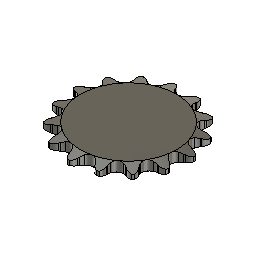
25Chain Sprocket Generator (Autodesk Fusion 360 design; units mm, degrees)
Autodesk Fusion 360 part; units mm, degrees
sketch "Teeth" plane through (0, 0, 0) normal (0, 0, 1) x (1, 0, 0)
  circle A0 centre (0, 0) radius 15.2709 construction
  line L0 (0, 15.2709) -> (-6.2112, 13.9507) construction
  arc A1 (-1.8813, 15.121) -> (-1.3133, 14.2074) centre (2.0529, 16.9333) ccw
  line L1 (-1.8813, 15.121) -> (-2.0352, 15.4552)
  arc A2 (-2.0352, 15.4552) -> (-3.2085, 16.7119) centre (-4.5218, 14.3098) ccw
  line L2 (0, 15.2709) -> (3.9262, 15.2709) construction
  line L3 (-1.8813, 15.121) -> (2.0529, 16.9333) construction
  line L4 (2.0529, 16.9333) -> (0, 15.2709) construction
  line L5 (0, 15.2709) -> (0, 0) construction
  arc A3 (-1.3133, 14.2074) -> (0, 13.581) centre (0, 15.2709) ccw
  arc A4 (3.2085, 16.7119) -> (2.0352, 15.4552) centre (4.5218, 14.3098) ccw
  line L6 (1.8813, 15.121) -> (2.0352, 15.4552)
  arc A5 (1.3133, 14.2074) -> (1.8813, 15.121) centre (-2.0529, 16.9333) ccw
  arc A6 (0, 13.581) -> (1.3133, 14.2074) centre (0, 15.2709) ccw
  arc A7 (-3.2085, 16.7119) -> (-3.5381, 16.6453) centre (0, 0) ccw
  arc A8 (3.5381, 16.6453) -> (3.2085, 16.7119) centre (0, 0) ccw
  circle A9 centre (0, 0) radius 17.0172
  dimension "d11" = 30.5418
  dimension "d12" = 6.35
  dimension "d14" = 39
  dimension "d15" = 14.267
  dimension "d16" = 2.6416
  dimension "d17" = 4.6228
  dimension "d18" = 1.6899
  dimension "d20" = 17.0172
  dimension "d50" = 34.0343
  constraint coincident A0.centre L5.end
  constraint coincident A0 L0.start
  constraint coincident A0 L0.end
  constraint vertical A0.centre L0.start
  constraint tangent A1 L1
  constraint tangent L1 A2
  constraint tangent A0 L2
  constraint horizontal L2
  constraint perpendicular L1 L3
  constraint coincident L0 A2.centre
  constraint coincident A1.centre L3.end
  constraint coincident L5 A3.end
  constraint coincident L0 L2.start
  constraint coincident L0.start L2.start
  constraint tangent A1 A3
  constraint symmetric A1.end L5 A5.start
  constraint symmetric A1.start L5 L6.start
  constraint symmetric A1 L5 A5
  constraint symmetric L1.end L5 A4.end
  constraint symmetric A2 L5 A4
  constraint symmetric L5 A3.end A6.start
  constraint symmetric L5 A3 A6
  constraint vertical A0.centre A3.end
  constraint symmetric L5 A2.end A4.start
  constraint symmetric L5 A7.end A8.start
  constraint symmetric L5 A7 A8
  constraint coincident A4.start A8.end
  measures "d11" diameter of A0
  measures "d12" distance of L0.start L0.end
  measures "d14" angle of L2 L4
  measures "d15" angle of L3 L4
  measures "d16" distance of A1.centre L0.start
  measures "d17" distance of A2.centre L0.start
  measures "d18" radius of A3
  measures "d20" radius of A7
  measures "d50" diameter of A9
extrude "Extrude1" add sketch "Teeth" along normal mid plane 2.794
extrude "Extrude3" cut sketch "Teeth" along normal through all and the other way through all contours A1 L1 A2 A3 A4 L6 A5 A6 A9
pattern_circular "C-Pattern1" count 15 over 360 about axis through (0, 0, 0) along (0, 0, 1) of "Extrude3"
sketch "Sketch4" plane through (0, 0, 0) normal (1, 0, 0) x (0, 1, 0)
  line L0 (-17.0172, 0.635) -> (-13.581, 1.397)
  line L1 (-13.581, 1.397) -> (0, 1.397)
  line L2 (-13.581, -1.397) -> (0, -1.397)
  line L3 (-17.0172, -0.635) -> (-13.581, -1.397)
  line L4 (0, 1.397) -> (0, -1.397)
  line L5 (-17.0172, 0.635) -> (-17.0172, -0.635)
  point P0 (-39.6283, 3.175)
  point P1 (-17.0172, 0)
  dimension "d54" = 2.794
  dimension "d55" = 17.0172
  dimension "d56" = 13.581
  dimension "d57" = 1.27
  constraint horizontal L1
  constraint horizontal L2
  constraint midpoint L4 origin
  constraint vertical L5
  constraint equal L1 L2
  constraint midpoint L5 P1
  constraint horizontal origin P1
  measures "d54" distance of L1.end L2.end
  measures "d55" distance of L4 L5
  measures "d56" distance of L2.end L2.start
  measures "d57" distance of L0.start L3.start
revolve "Revolve1" cut sketch "Sketch4" angle 360 about axis through (0, 0, 1.75) along (0, 0, 1) keep common part
equation "p = 0.25 in" comment "0.25 for #25, 0.375 for #35"
equation "Dr = 0.13 in" comment "0.13 for #25, 0.2 for #35"
equation "Ds = 1.0005 * Dr + 0.003 in"
equation "n = 15" comment "Number of Teeth"
equation "PD = p / sin(( 180 / n ) * 1 deg)"
equation "A_angle = 35 deg + ( 60 / n ) * 1 deg"
equation "B_angle = 18 deg - ( 56 / n ) * 1 deg"
equation "ac = 0.8 * Dr"
equation "ab = 1.4 * Dr"
equation "OD = PD + 0.55 * p"
equation "d11 = PD"
equation "d12 = p"
equation "d14 = A_angle"
equation "d15 = B_angle"
equation "d16 = ac"
equation "d17 = ab"
equation "d18 = Ds / 2"
equation "d20 = OD / 2"
equation "d50 = OD"
equation "d52 = n"
equation "d55 = OD / 2"
equation "d56 = ( PD - Ds ) / 2"
